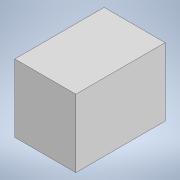
# Autodesk Inventor part: Inventor2020test
Saved by Autodesk Inventor 2020.3 (Build 243373010, 373A)
## iProperties
Created: 2020-11-02
Part Number: Inventor2020test
Material: Generic
Document SubType Name: Modeling
Designer: smccaffrey
Density: 1 g/cm^3
Appearance: Default
Author: smccaffrey
Autodesk Inventor part; units mm, degrees
ref_plane "YZ Plane" through (0, 0, 0) normal (1, 0, 0) x (0, 1, 0)
ref_plane "XZ Plane" through (0, 0, 0) normal (0, 1, 0) x (-1, 0, 0)
ref_plane "XY Plane" through (0, 0, 0) normal (0, 0, 1) x (1, 0, 0)
sketch "Sketch1" plane through (0, 0, 0) normal (0, 1, 0) x (-1, 0, 0)
  line L0 (0.3033, 0) -> (23.1491, 0)
  line L1 (23.1491, 0) -> (23.1491, -33.4004)
  line L2 (23.1491, -33.4004) -> (0.3033, -33.4004)
  line L3 (0.3033, -33.4004) -> (0.3033, 0)
  point P0 (0, 0)
  constraints: 8 end point, 2 parallel, 1 horizontal, 1 perpendicular
extrude "Extrusion1" add sketch "Sketch1" along normal blind 25.4
body "Solid1"
